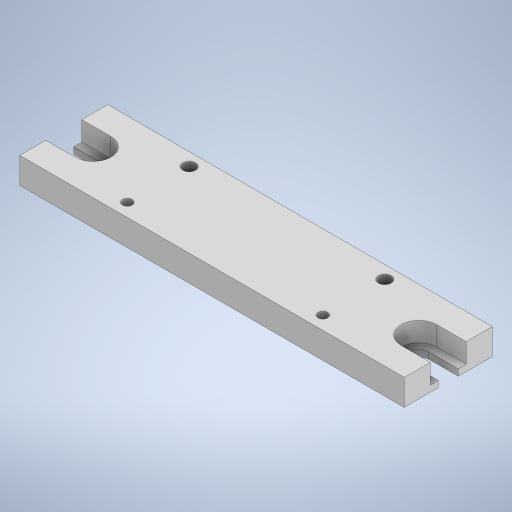
# Autodesk Inventor part: Base Laser distintas
Saved by Autodesk Inventor 2023 (Build 270158000, 158)
## iProperties
Created: 2023-01-13
Part Number: Base Laser distintas
Material: Generic
Document SubType Name: Modeling
Designer: Ruth
Density: 1 g/cm^3
Appearance: Default
Author: Ruth
## iProperties of the stored document Base Laser_3DPrint.ipt
Created: 2023-01-16
Part Number: Base Laser_3DPrint
Material: Generic
Document SubType Name: Modeling
Designer: Ruth
Density: 1 g/cm^3
Appearance: Default
Author: Ruth
Autodesk Inventor part; units mm, degrees
ref_plane "YZ Plane" through (0, 0, 0) normal (1, 0, 0) x (0, 1, 0)
ref_plane "XZ Plane" through (0, 0, 0) normal (0, 1, 0) x (-1, 0, 0)
ref_plane "XY Plane" through (0, 0, 0) normal (0, 0, 1) x (1, 0, 0)
sketch "Sketch1" plane through (0, 0, 0) normal (0, 1, 0) x (-1, 0, 0)
  circle A0 centre (118.5461, -28.7809) radius 1.975
  circle A1 centre (118.5461, -9.7809) radius 1.49
  arc A2 (138.5461, -13.7809) -> (138.5461, -24.7809) centre (138.5461, -19.2809) ccw
  circle A3 centre (58.5461, -28.8073) radius 1.975
  line L0 (147.5461, -32.7809) -> (29.5461, -32.7809)
  line L1 (29.5461, -5.7809) -> (147.5461, -5.7809)
  arc A4 (38.5461, -24.7809) -> (38.5461, -13.7809) centre (38.5461, -19.2809) ccw
  line L2 (29.5461, -32.7809) -> (29.5461, -5.7809)
  circle A5 centre (58.5461, -9.8073) radius 1.49
  arc A6 (138.5461, -16.2059) -> (138.5461, -22.3559) centre (138.5461, -19.2809) ccw
  arc A7 (38.5461, -22.3559) -> (38.5461, -16.2059) centre (38.5461, -19.2809) ccw
  line L3 (143.1062, -22.3559) -> (147.5461, -22.3559)
  line L4 (143.1062, -16.2059) -> (147.5461, -16.2059)
  line L5 (147.5461, -32.7809) -> (147.5461, -22.3559)
  line L6 (147.5461, -16.2059) -> (147.5461, -5.7809)
  line L7 (143.1062, -22.3559) -> (138.5461, -22.3559)
  line L8 (143.1062, -16.2059) -> (138.5461, -16.2059)
  line L9 (138.5461, -24.7809) -> (147.5461, -24.7809)
  line L10 (138.5461, -13.7809) -> (147.5461, -13.7809)
  line L11 (38.5461, -22.3559) -> (29.5461, -22.3559)
  line L12 (38.5461, -24.7809) -> (29.5461, -24.7809)
  line L13 (38.5461, -16.2059) -> (29.5461, -16.2059)
  line L14 (38.5461, -13.7809) -> (29.5461, -13.7809)
  point P0 (88.5461, -32.7809)
  point P1 (88.5461, -5.7809)
  dimension "d162" = 60
  dimension "d163" = 60
  dimension "d165" = 100
  dimension "d183" = 11
  dimension "d184" = 11
  dimension "d185" = 6.15
  dimension "d186" = 6.15
  dimension "d187" = 3.95
  dimension "d188" = 2.98
  dimension "d189" = 3.95
  dimension "d190" = 2.98
  dimension "d202" = 9
  dimension "d203" = 9
  dimension "d204" = 9
  dimension "d212" = 19
  dimension "d213" = 19
  dimension "d214" = 27
  dimension "d215" = 4
  dimension "d216" = 4
  dimension "d217" = 13.5
  dimension "d218" = 30
  dimension "d219" = 30
  constraints: 30 end point, 10 perpendicular, 8 centre point, 8 point on circle, 6 point on line, 2 coincident, 2 horizontal, 2 midpoint, 2 parallel, 1 tangent
  measures "d162" distance of A3.centre A0.centre
  measures "d163" distance of A5.centre A1.centre
  measures "d165" distance of A4.centre A2.centre
  measures "d183" diameter of A2
  measures "d184" diameter of A4
  measures "d185" diameter of A6
  measures "d186" diameter of A7
  measures "d187" diameter of A0
  measures "d188" diameter of A1
  measures "d189" diameter of A3
  measures "d190" diameter of A5
  measures "d202" distance from line of L2 A4.centre
  measures "d203" distance from line of A2.centre L5
  measures "d204" distance from line of L6 A2.centre
  measures "d212" distance of A5.centre A3.centre
  measures "d213" distance of A1.centre A0.centre
  measures "d214" distance of L0.end L1.start
  measures "d215" distance from line of L0 A0.centre
  measures "d216" distance from line of L1 A1.centre
  measures "d217" distance from line of L1 A2.centre
  measures "d218" horizontal distance of A3.centre point (88.546, -32.781)
  measures "d219" horizontal distance of A5.centre point (88.546, -5.781)
extrude "Extrusion13" add sketch "Sketch1" along normal blind 8 contours A2 L9 L5 L0 L2 L12 A4 L14 L1 L6 L10
extrude "Extrusion14" add sketch "Sketch1" along normal blind 2 contours L14 A4 L12 L2 L11 A7 L13
extrude "Extrusion15" add sketch "Sketch1" along normal blind 2 contours L10 L6 L4 L8 A6 L7 L3 L5 L9 A2
body "Solid3"
